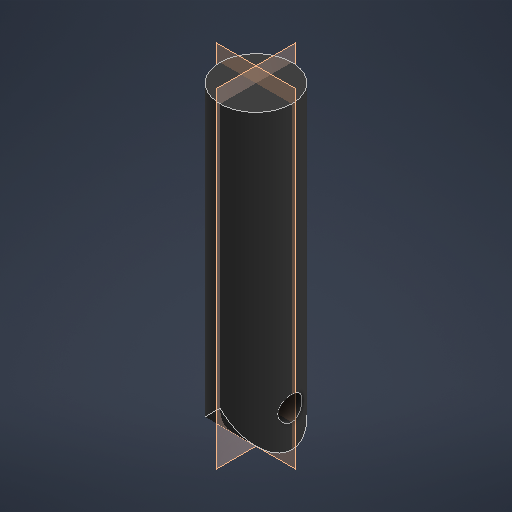
# Autodesk Inventor part: Camera Encasing
Saved by Autodesk Inventor 2026.2 (Build 302298010, 298A)
## iProperties
Created: 2026-04-01
Part Number: Camera Encasing
Material: Rubber
Document SubType Name: Modeling
Designer: piete
Density: 0.93 g/cm^3
Appearance: Rubber - Black
Author: piete
Autodesk Inventor part; units mm, degrees
ref_plane "XZ Plane" through (0, 0, 0) normal (0, 1, 0) x (-1, 0, 0)
sketch "Sketch1" plane through (0, 0, 0) normal (0, 1, 0) x (-1, 0, 0)
  circle A0 centre (0, 0) radius 3
  dimension "d0" = 6
  constraints: 1 centre point, 1 coincident
  measures "d0" diameter of A0
extrude "Extrusion1" add sketch "Sketch1" along normal blind 25
sketch "Sketch2" plane through (0, 0, 0) normal (1, 0, 0) x (0, 1, 0)
  circle A0 centre (3, 0) radius 1
  line L0 (0, -3) -> (0, 3) projected
  circle A1 centre (3, 0) radius 3
  line L1 (3, 3) -> (0, 3)
  line L2 (0, 3) -> (25, 3) projected
  line L3 (0, 3) -> (0, -3)
  line L4 (3, -3) -> (0, -3)
  point P0 (0, 0)
  point P1 (0, 0)
  dimension "d3" = 2
  dimension "d4" = 3
  dimension "d5" = 3
  dimension "d6" = 6
  constraints: 6 end point, 2 centre point, 2 point on circle, 1 coincident, 1 collinear, 1 perpendicular, 1 tangent
  measures "d3" diameter of A0
  measures "d4" distance from line of L0 A0.centre
  measures "d5" horizontal distance of L0.start A0.centre
  measures "d6" diameter of A1
extrude "Extrusion2" cut sketch "Sketch2" along normal through all both and the other way through all contours A0 | L0 A1 L4 | L0 L1 A1
body "Solid1"
